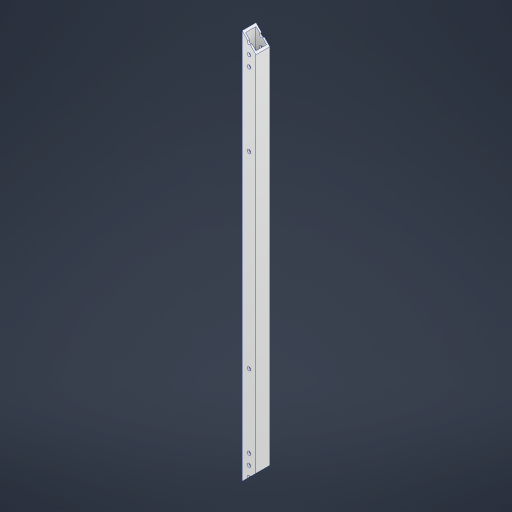
# Autodesk Inventor part: STRU_003_BilletPole_28in_Angled
Saved by Autodesk Inventor 2024.2 (Build 282272000, 272)
## iProperties
Created: 2024-07-23
Part Number: STRU_003_BilletPole_28in_Angled
Material: Aluminum 6061
Document SubType Name: Modeling
Designer: bryan
Density: 2.7 g/cm^3
Appearance: Aluminum - Flat
Mass: 518.66 g
Surface Area: 1226.29 cm^2
Volume: 192.096 cm^3
Author: bryan
Autodesk Inventor part; units mm, degrees
ref_plane "YZ Plane" through (0, 0, 0) normal (1, 0, 0) x (0, 1, 0)
ref_plane "XZ Plane" through (0, 0, 0) normal (0, 1, 0) x (-1, 0, 0)
ref_plane "XY Plane" through (0, 0, 0) normal (0, 0, 1) x (1, 0, 0)
sketch "Sketch1" plane through (0, 0, 0) normal (0, 1, 0) x (-1, 0, 0)
  line L0 (-12.7, -12.7) -> (12.7, -12.7)
  line L1 (12.7, -12.7) -> (12.7, 12.7)
  line L2 (12.7, 12.7) -> (-12.7, 12.7)
  line L3 (-12.7, 12.7) -> (-12.7, -12.7)
  line L4 (-12.7, -12.7) -> (12.7, 12.7) construction
  line L5 (12.7, -12.7) -> (-12.7, 12.7) construction
  line L6 (9.525, 9.525) -> (9.525, -9.525)
  line L7 (9.525, -9.525) -> (-9.525, -9.525)
  line L8 (-9.525, -9.525) -> (-9.525, 9.525)
  line L9 (-9.525, 9.525) -> (9.525, 9.525)
  point P0 (0, 0)
  dimension "d0" = 25.4
  dimension "d1" = 25.4
  dimension "d2" = 3.175
  constraints: 20 end point, 4 parallel, 2 midpoint, 2 perpendicular, 1 horizontal, 3 other
  measures "d0" distance of L2.end L1.end
  measures "d1" distance of L1.end L0.end
  measures "d2" distance between parallel lines of L1 L6
extrude "Extrusion1" add sketch "Sketch1" along normal mid plane 711.2
sketch "Sketch2" plane through (-12.7, 355.6, 12.7) normal (0, 0, 1) x (1, 0, 0)
  line L0 (0, 0) -> (25.4, 0) projected
  line L1 (0, 0) -> (25.4, -25.4)
  line L2 (25.4, -711.2) -> (25.4, 0) projected
  circle A0 centre (12.7, -31.75) radius 3.2512
  circle A1 centre (12.7, -50.8) radius 3.2512
  line L3 (0, -711.2) -> (0, 0) projected
  line L4 (0, -355.6) -> (25.4, -355.6) construction
  line L5 (0, -711.2) -> (25.4, -711.2)
  line L6 (0, -711.2) -> (25.4, -685.8)
  circle A2 centre (12.7, -679.45) radius 3.2512
  circle A3 centre (12.7, -660.4) radius 3.2512
  circle A4 centre (12.7, -12.7) radius 3.2512
  circle A5 centre (12.7, -698.5) radius 3.2512
  point P0 (12.7, -355.6)
  point P1 (12.7, 0)
  point P2 (12.7, -711.2)
  point P3 (14.9989, -14.9989)
  point P4 (10.4011, -10.4011)
  point P5 (14.9989, -696.2011)
  point P6 (10.4011, -700.7989)
  dimension "d5" = 25.4
  dimension "d6" = 6.5024
  dimension "d7" = 31.75
  dimension "d8" = 19.05
  constraints: 8 end point, 6 centre point, 5 midpoint, 4 symmetric about line, 3 equal radius, 2 vertical alignment, 1 point on line, 2 other
  measures "d5" distance of L0.end L1.end
  measures "d6" diameter of A0
  measures "d7" distance from line of L0 A0.centre
  measures "d8" distance of A1.centre A0.centre
extrude "Extrusion2" cut sketch "Sketch2" against normal blind 711.2 contours L0 L2 L1 A4 | A4 L1 | L1 A4 | L6 A5 L2 L5 | A5 L6 | L6 A5 | A0 | A1 | A2 | A3
sketch "Sketch3" plane through (-12.7, -355.6, 12.7) normal (0, 0, 1) x (1, 0, 0)
  line L0 (0, 711.2) -> (0, 0) construction
  line L1 (0, 355.6) -> (25.4, 355.6) construction
  line L2 (25.4, 25.4) -> (25.4, 685.8) construction
  circle A0 centre (12.7, 184.15) radius 3.2512
  circle A1 centre (12.7, 527.05) radius 3.2512
  point P0 (12.7, 355.6)
  dimension "d14" = 6.5024
  dimension "d15" = 171.45
  dimension "d16" = 158.75
  constraints: 3 midpoint, 2 centre point, 2 end point, 1 equal radius, 1 vertical alignment, 1 other
  measures "d14" diameter of A0
  measures "d15" distance from line of L1 A0.centre
  measures "d16" vertical distance of A0.centre L2.start
extrude "Extrusion3" cut sketch "Sketch3" against normal blind 25.4
body "Solid1"
